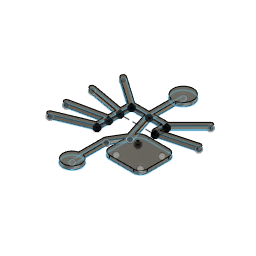
2023_04_27_Conductive Pla v3 (Autodesk Fusion 360 design; units mm, degrees)
Autodesk Fusion 360 part; units mm, degrees
note: some values were not read from the file. Chosen so that the rebuilt part matches the saved one: which bodies a step acts on. Set by a fixed rule: which sketch regions a step uses.
sketch "Sketch1" plane through (0, 0, 0) normal (0, 0, 1) x (1, 0, 0)
  line L0 (0, 0) -> (1.75, 0)
  line L1 (1.75, 0) -> (1.75, 100)
  line L2 (1.75, 100) -> (0, 100)
  line L3 (0, 100) -> (0, 0)
  line L4 (4.7368, 100) -> (4.7368, 0)
  line L5 (4.7368, 0) -> (6.4868, 0)
  line L6 (6.4868, 100) -> (4.7368, 100)
  line L7 (6.4868, 0) -> (6.4868, 100)
  line L8 (9.4737, 100) -> (9.4737, 0)
  line L9 (9.4737, 0) -> (11.2237, 0)
  line L10 (11.2237, 100) -> (9.4737, 100)
  line L11 (11.2237, 0) -> (11.2237, 100)
  line L12 (14.2105, 100) -> (14.2105, 0)
  line L13 (14.2105, 0) -> (15.9605, 0)
  line L14 (15.9605, 100) -> (14.2105, 100)
  line L15 (15.9605, 0) -> (15.9605, 100)
  line L16 (18.9474, 100) -> (18.9474, 0)
  line L17 (18.9474, 0) -> (20.6974, 0)
  line L18 (20.6974, 100) -> (18.9474, 100)
  line L19 (20.6974, 0) -> (20.6974, 100)
  line L20 (23.6842, 100) -> (23.6842, 0)
  line L21 (23.6842, 0) -> (25.4342, 0)
  line L22 (25.4342, 100) -> (23.6842, 100)
  line L23 (25.4342, 0) -> (25.4342, 100)
  line L24 (28.4211, 100) -> (28.4211, 0)
  line L25 (28.4211, 0) -> (30.1711, 0)
  line L26 (30.1711, 100) -> (28.4211, 100)
  line L27 (30.1711, 0) -> (30.1711, 100)
  line L28 (33.1579, 100) -> (33.1579, 0)
  line L29 (33.1579, 0) -> (34.9079, 0)
  line L30 (34.9079, 100) -> (33.1579, 100)
  line L31 (34.9079, 0) -> (34.9079, 100)
  line L32 (37.8947, 100) -> (37.8947, 0)
  line L33 (37.8947, 0) -> (39.6447, 0)
  line L34 (39.6447, 100) -> (37.8947, 100)
  line L35 (39.6447, 0) -> (39.6447, 100)
  line L36 (42.6316, 100) -> (42.6316, 0)
  line L37 (42.6316, 0) -> (44.3816, 0)
  line L38 (44.3816, 100) -> (42.6316, 100)
  line L39 (44.3816, 0) -> (44.3816, 100)
  line L40 (47.3684, 100) -> (47.3684, 0)
  line L41 (47.3684, 0) -> (49.1184, 0)
  line L42 (49.1184, 100) -> (47.3684, 100)
  line L43 (49.1184, 0) -> (49.1184, 100)
  line L44 (52.1053, 100) -> (52.1053, 0)
  line L45 (52.1053, 0) -> (53.8553, 0)
  line L46 (53.8553, 100) -> (52.1053, 100)
  line L47 (53.8553, 0) -> (53.8553, 100)
  line L48 (56.8421, 100) -> (56.8421, 0)
  line L49 (56.8421, 0) -> (58.5921, 0)
  line L50 (58.5921, 100) -> (56.8421, 100)
  line L51 (58.5921, 0) -> (58.5921, 100)
  line L52 (61.5789, 100) -> (61.5789, 0)
  line L53 (61.5789, 0) -> (63.3289, 0)
  line L54 (63.3289, 100) -> (61.5789, 100)
  line L55 (63.3289, 0) -> (63.3289, 100)
  line L56 (66.3158, 100) -> (66.3158, 0)
  line L57 (66.3158, 0) -> (68.0658, 0)
  line L58 (68.0658, 100) -> (66.3158, 100)
  line L59 (68.0658, 0) -> (68.0658, 100)
  line L60 (71.0526, 100) -> (71.0526, 0)
  line L61 (71.0526, 0) -> (72.8026, 0)
  line L62 (72.8026, 100) -> (71.0526, 100)
  line L63 (72.8026, 0) -> (72.8026, 100)
  line L64 (75.7895, 100) -> (75.7895, 0)
  line L65 (75.7895, 0) -> (77.5395, 0)
  line L66 (77.5395, 100) -> (75.7895, 100)
  line L67 (77.5395, 0) -> (77.5395, 100)
  line L68 (80.5263, 100) -> (80.5263, 0)
  line L69 (80.5263, 0) -> (82.2763, 0)
  line L70 (82.2763, 100) -> (80.5263, 100)
  line L71 (82.2763, 0) -> (82.2763, 100)
  line L72 (85.2632, 100) -> (85.2632, 0)
  line L73 (85.2632, 0) -> (87.0132, 0)
  line L74 (87.0132, 100) -> (85.2632, 100)
  line L75 (87.0132, 0) -> (87.0132, 100)
  line L76 (90, 100) -> (90, 0)
  line L77 (90, 0) -> (91.75, 0)
  line L78 (91.75, 100) -> (90, 100)
  line L79 (91.75, 0) -> (91.75, 100)
  line L80 (0, 100) -> (6.4868, 100)
  line L81 (6.4868, 100) -> (6.4868, 97.0952)
  line L82 (6.4868, 97.0952) -> (0, 97.0952)
  line L83 (0, 97.0952) -> (0, 100)
  line L84 (4.7368, 0) -> (11.2237, 0)
  line L85 (11.2237, 0) -> (11.2237, 2.7697)
  line L86 (11.2237, 2.7697) -> (4.7368, 2.7697)
  line L87 (4.7368, 2.7697) -> (4.7368, 0)
  line L88 (9.5, 100) -> (15.9868, 100)
  line L89 (15.9868, 100) -> (15.9868, 97.0952)
  line L90 (9.5, 97.0952) -> (9.5, 100)
  line L91 (15.9868, 97.0952) -> (9.5, 97.0952)
  line L92 (14.2368, 0) -> (20.7237, 0)
  line L93 (20.7237, 0) -> (20.7237, 2.7697)
  line L94 (14.2368, 2.7697) -> (14.2368, 0)
  line L95 (20.7237, 2.7697) -> (14.2368, 2.7697)
  line L96 (19, 100) -> (25.4868, 100)
  line L97 (25.4868, 100) -> (25.4868, 97.0952)
  line L98 (19, 97.0952) -> (19, 100)
  line L99 (25.4868, 97.0952) -> (19, 97.0952)
  line L100 (23.7368, 0) -> (30.2237, 0)
  line L101 (30.2237, 0) -> (30.2237, 2.7697)
  line L102 (23.7368, 2.7697) -> (23.7368, 0)
  line L103 (30.2237, 2.7697) -> (23.7368, 2.7697)
  line L104 (28.5, 100) -> (34.9868, 100)
  line L105 (34.9868, 100) -> (34.9868, 97.0952)
  line L106 (28.5, 97.0952) -> (28.5, 100)
  line L107 (34.9868, 97.0952) -> (28.5, 97.0952)
  line L108 (33.2368, 0) -> (39.7237, 0)
  line L109 (39.7237, 0) -> (39.7237, 2.7697)
  line L110 (33.2368, 2.7697) -> (33.2368, 0)
  line L111 (39.7237, 2.7697) -> (33.2368, 2.7697)
  line L112 (38, 100) -> (44.4868, 100)
  line L113 (44.4868, 100) -> (44.4868, 97.0952)
  line L114 (38, 97.0952) -> (38, 100)
  line L115 (44.4868, 97.0952) -> (38, 97.0952)
  line L116 (42.7368, 0) -> (49.2237, 0)
  line L117 (49.2237, 0) -> (49.2237, 2.7697)
  line L118 (42.7368, 2.7697) -> (42.7368, 0)
  line L119 (49.2237, 2.7697) -> (42.7368, 2.7697)
  line L120 (47.5, 100) -> (53.9868, 100)
  line L121 (53.9868, 100) -> (53.9868, 97.0952)
  line L122 (47.5, 97.0952) -> (47.5, 100)
  line L123 (53.9868, 97.0952) -> (47.5, 97.0952)
  line L124 (52.2368, 0) -> (58.7237, 0)
  line L125 (58.7237, 0) -> (58.7237, 2.7697)
  line L126 (52.2368, 2.7697) -> (52.2368, 0)
  line L127 (58.7237, 2.7697) -> (52.2368, 2.7697)
  line L128 (57, 100) -> (63.4868, 100)
  line L129 (63.4868, 100) -> (63.4868, 97.0952)
  line L130 (57, 97.0952) -> (57, 100)
  line L131 (63.4868, 97.0952) -> (57, 97.0952)
  line L132 (61.7368, 0) -> (68.2237, 0)
  line L133 (68.2237, 0) -> (68.2237, 2.7697)
  line L134 (61.7368, 2.7697) -> (61.7368, 0)
  line L135 (68.2237, 2.7697) -> (61.7368, 2.7697)
  line L136 (66.5, 100) -> (72.9868, 100)
  line L137 (72.9868, 100) -> (72.9868, 97.0952)
  line L138 (66.5, 97.0952) -> (66.5, 100)
  line L139 (72.9868, 97.0952) -> (66.5, 97.0952)
  line L140 (71.2368, 0) -> (77.7237, 0)
  line L141 (77.7237, 0) -> (77.7237, 2.7697)
  line L142 (71.2368, 2.7697) -> (71.2368, 0)
  line L143 (77.7237, 2.7697) -> (71.2368, 2.7697)
  line L144 (76, 100) -> (82.4868, 100)
  line L145 (82.4868, 100) -> (82.4868, 97.0952)
  line L146 (76, 97.0952) -> (76, 100)
  line L147 (82.4868, 97.0952) -> (76, 97.0952)
  line L148 (80.7368, 0) -> (87.2237, 0)
  line L149 (87.2237, 0) -> (87.2237, 2.7697)
  line L150 (80.7368, 2.7697) -> (80.7368, 0)
  line L151 (87.2237, 2.7697) -> (80.7368, 2.7697)
  line L152 (85.5, 100) -> (91.9868, 100)
  line L153 (91.9868, 100) -> (91.9868, 97.0952)
  line L154 (85.5, 97.0952) -> (85.5, 100)
  line L155 (91.9868, 97.0952) -> (85.5, 97.0952)
  line L156 (90.2368, 0) -> (96.7237, 0)
  line L157 (96.7237, 0) -> (96.7237, 2.7697)
  line L158 (90.2368, 2.7697) -> (90.2368, 0)
  line L159 (96.7237, 2.7697) -> (90.2368, 2.7697)
  line L160 (109.2368, 2.7697) -> (109.2368, 0)
  line L161 (182.0132, 0) -> (182.0132, 100)
  line L162 (170.7895, 100) -> (170.7895, 0)
  line L163 (147.2368, 2.7697) -> (147.2368, 0)
  line L164 (134.6447, 100) -> (132.8947, 100)
  line L165 (153.5921, 0) -> (153.5921, 100)
  line L166 (125.2237, 0) -> (125.2237, 2.7697)
  line L167 (147.2368, 0) -> (153.7237, 0)
  line L168 (166.0526, 100) -> (166.0526, 0)
  line L169 (180.2632, 100) -> (180.2632, 0)
  line L170 (115.6974, 0) -> (115.6974, 100)
  line L171 (185, 0) -> (186.75, 0)
  line L172 (118.7368, 0) -> (125.2237, 0)
  line L173 (96.75, 0) -> (96.75, 100)
  line L174 (120.4342, 0) -> (120.4342, 100)
  line L175 (115.6974, 100) -> (113.9474, 100)
  line L176 (128.2368, 2.7697) -> (128.2368, 0)
  line L177 (139.4868, 97.0952) -> (133, 97.0952)
  line L178 (109.2368, 0) -> (115.7237, 0)
  line L179 (128.1579, 100) -> (128.1579, 0)
  line L180 (161.3158, 100) -> (161.3158, 0)
  line L181 (144.1184, 0) -> (144.1184, 100)
  line L182 (166.2368, 0) -> (172.7237, 0)
  line L183 (170.7895, 0) -> (172.5395, 0)
  line L184 (113.9474, 0) -> (115.6974, 0)
  line L185 (134.7237, 2.7697) -> (128.2368, 2.7697)
  line L186 (163.0658, 0) -> (163.0658, 100)
  line L187 (148.8553, 0) -> (148.8553, 100)
  line L188 (172.7237, 0) -> (172.7237, 2.7697)
  line L189 (99.7368, 0) -> (101.4868, 0)
  line L190 (144.2237, 0) -> (144.2237, 2.7697)
  line L191 (137.6316, 0) -> (139.3816, 0)
  line L192 (137.7368, 2.7697) -> (137.7368, 0)
  line L193 (153.7237, 0) -> (153.7237, 2.7697)
  line L194 (175.5263, 0) -> (177.2763, 0)
  line L195 (120.4868, 100) -> (120.4868, 97.0952)
  line L196 (139.3816, 0) -> (139.3816, 100)
  line L197 (186.75, 0) -> (186.75, 100)
  line L198 (177.2763, 0) -> (177.2763, 100)
  line L199 (156.5789, 100) -> (156.5789, 0)
  line L200 (125.1711, 0) -> (125.1711, 100)
  line L201 (95, 97.0952) -> (95, 100)
  line L202 (123.4211, 100) -> (123.4211, 0)
  line L203 (158.3289, 0) -> (158.3289, 100)
  line L204 (104.4737, 0) -> (106.2237, 0)
  line L205 (156.5789, 0) -> (158.3289, 0)
  line L206 (147.1053, 100) -> (147.1053, 0)
  line L207 (123.4211, 0) -> (125.1711, 0)
  line L208 (175.7368, 2.7697) -> (175.7368, 0)
  line L209 (175.7368, 0) -> (182.2237, 0)
  line L210 (175.5263, 100) -> (175.5263, 0)
  line L211 (182.2237, 0) -> (182.2237, 2.7697)
  line L212 (104.5, 100) -> (110.9868, 100)
  line L213 (180.2632, 0) -> (182.0132, 0)
  line L214 (128.1579, 0) -> (129.9079, 0)
  line L215 (137.6316, 100) -> (137.6316, 0)
  line L216 (177.4868, 97.0952) -> (171, 97.0952)
  line L217 (110.9868, 97.0952) -> (104.5, 97.0952)
  line L218 (95, 0) -> (96.75, 0)
  line L219 (99.7368, 0) -> (106.2237, 0)
  line L220 (161.5, 100) -> (167.9868, 100)
  line L221 (110.9868, 100) -> (110.9868, 97.0952)
  line L222 (156.7368, 2.7697) -> (156.7368, 0)
  line L223 (163.2237, 2.7697) -> (156.7368, 2.7697)
  line L224 (153.7237, 2.7697) -> (147.2368, 2.7697)
  line L225 (142.3684, 0) -> (144.1184, 0)
  line L226 (185, 100) -> (185, 0)
  line L227 (104.4737, 100) -> (104.4737, 0)
  line L228 (99.7368, 100) -> (99.7368, 0)
  line L229 (166.0526, 0) -> (167.8026, 0)
  line L230 (180.5, 97.0952) -> (180.5, 100)
  line L231 (156.7368, 0) -> (163.2237, 0)
  line L232 (172.5395, 0) -> (172.5395, 100)
  line L233 (134.7237, 0) -> (134.7237, 2.7697)
  line L234 (185.2368, 0) -> (191.7237, 0)
  line L235 (120.4868, 97.0952) -> (114, 97.0952)
  line L236 (185.2368, 2.7697) -> (185.2368, 0)
  line L237 (172.7237, 2.7697) -> (166.2368, 2.7697)
  line L238 (167.9868, 100) -> (167.9868, 97.0952)
  line L239 (142.3684, 100) -> (142.3684, 0)
  line L240 (101.4868, 100) -> (99.7368, 100)
  line L241 (151.8421, 100) -> (151.8421, 0)
  line L242 (147.1053, 0) -> (148.8553, 0)
  line L243 (133, 100) -> (139.4868, 100)
  line L244 (167.9868, 97.0952) -> (161.5, 97.0952)
  line L245 (163.2237, 0) -> (163.2237, 2.7697)
  line L246 (132.8947, 0) -> (134.6447, 0)
  line L247 (129.9868, 100) -> (129.9868, 97.0952)
  line L248 (118.7368, 2.7697) -> (118.7368, 0)
  line L249 (151.8421, 0) -> (153.5921, 0)
  line L250 (109.2105, 100) -> (109.2105, 0)
  line L251 (158.3289, 100) -> (156.5789, 100)
  line L252 (132.8947, 100) -> (132.8947, 0)
  line L253 (118.6842, 0) -> (120.4342, 0)
  line L254 (95, 100) -> (95, 0)
  line L255 (115.7237, 0) -> (115.7237, 2.7697)
  line L256 (118.6842, 100) -> (118.6842, 0)
  line L257 (106.2237, 0) -> (106.2237, 2.7697)
  line L258 (125.1711, 100) -> (123.4211, 100)
  line L259 (113.9474, 100) -> (113.9474, 0)
  line L260 (101.4868, 0) -> (101.4868, 100)
  line L261 (128.2368, 0) -> (134.7237, 0)
  line L262 (106.2237, 0) -> (106.2237, 100)
  line L263 (134.6447, 0) -> (134.6447, 100)
  line L264 (110.9605, 0) -> (110.9605, 100)
  line L265 (96.75, 100) -> (95, 100)
  line L266 (106.2237, 100) -> (104.4737, 100)
  line L267 (99.7368, 2.7697) -> (99.7368, 0)
  line L268 (110.9605, 100) -> (109.2105, 100)
  line L269 (129.9079, 100) -> (128.1579, 100)
  line L270 (158.4868, 97.0952) -> (152, 97.0952)
  line L271 (142.5, 100) -> (148.9868, 100)
  line L272 (180.5, 100) -> (186.9868, 100)
  line L273 (182.0132, 100) -> (180.2632, 100)
  line L274 (166.2368, 2.7697) -> (166.2368, 0)
  line L275 (144.1184, 100) -> (142.3684, 100)
  line L276 (139.4868, 100) -> (139.4868, 97.0952)
  line L277 (106.2237, 2.7697) -> (99.7368, 2.7697)
  line L278 (104.5, 97.0952) -> (104.5, 100)
  line L279 (167.8026, 100) -> (166.0526, 100)
  line L280 (191.7237, 2.7697) -> (185.2368, 2.7697)
  line L281 (182.2237, 2.7697) -> (175.7368, 2.7697)
  line L282 (161.5, 97.0952) -> (161.5, 100)
  line L283 (144.2237, 2.7697) -> (137.7368, 2.7697)
  line L284 (137.7368, 0) -> (144.2237, 0)
  line L285 (142.5, 97.0952) -> (142.5, 100)
  line L286 (133, 97.0952) -> (133, 100)
  line L287 (186.9868, 97.0952) -> (180.5, 97.0952)
  line L288 (177.4868, 100) -> (177.4868, 97.0952)
  line L289 (171, 100) -> (177.4868, 100)
  line L290 (123.5, 100) -> (129.9868, 100)
  line L291 (114, 100) -> (120.4868, 100)
  line L292 (158.4868, 100) -> (158.4868, 97.0952)
  line L293 (148.9868, 97.0952) -> (142.5, 97.0952)
  line L294 (120.4342, 100) -> (118.6842, 100)
  line L295 (129.9868, 97.0952) -> (123.5, 97.0952)
  line L296 (101.4868, 100) -> (101.4868, 97.0952)
  line L297 (114, 97.0952) -> (114, 100)
  line L298 (167.8026, 0) -> (167.8026, 100)
  line L299 (161.3158, 0) -> (163.0658, 0)
  line L300 (186.75, 100) -> (185, 100)
  line L301 (95, 100) -> (101.4868, 100)
  line L302 (101.4868, 97.0952) -> (95, 97.0952)
  line L303 (148.8553, 100) -> (147.1053, 100)
  line L304 (153.5921, 100) -> (151.8421, 100)
  line L305 (172.5395, 100) -> (170.7895, 100)
  line L306 (123.5, 97.0952) -> (123.5, 100)
  line L307 (115.7237, 2.7697) -> (109.2368, 2.7697)
  line L308 (191.7237, 0) -> (191.7237, 2.7697)
  line L309 (177.2763, 100) -> (175.5263, 100)
  line L310 (148.9868, 100) -> (148.9868, 97.0952)
  line L311 (125.2237, 2.7697) -> (118.7368, 2.7697)
  line L312 (139.3816, 100) -> (137.6316, 100)
  line L313 (152, 100) -> (158.4868, 100)
  line L314 (109.2105, 0) -> (110.9605, 0)
  line L315 (129.9079, 0) -> (129.9079, 100)
  line L316 (186.9868, 100) -> (186.9868, 97.0952)
  line L317 (152, 97.0952) -> (152, 100)
  line L318 (171, 97.0952) -> (171, 100)
  line L319 (163.0658, 100) -> (161.3158, 100)
  point P0 (95, 0)
  dimension "d1" = 1.75
  dimension "d2" = 100
  dimension "d5" = 90
  dimension "d6" = 0
  dimension "d9" = 9.5
  dimension "d10" = 0
  dimension "d13" = 90
  dimension "d14" = 0
  dimension "d17" = 9.5
  dimension "d18" = 0
  dimension "d19" = 1.75
  dimension "d20" = 100
  constraint horizontal L0
  constraint vertical L1
  constraint horizontal L2
  constraint vertical L3
  constraint coincident L0.start L3.end
  constraint horizontal L80
  constraint vertical L81
  constraint horizontal L82
  constraint vertical L83
  constraint coincident L7 L81.end
  constraint horizontal L84
  constraint vertical L85
  constraint horizontal L86
  constraint vertical L87
  constraint coincident L11 L85.end
  constraint horizontal L218
  constraint vertical L173
  constraint horizontal L265
  constraint vertical L254
  constraint coincident P0 L218.start
  constraint horizontal L301
  constraint vertical L296
  constraint horizontal L302
  constraint vertical L201
  constraint coincident L296.end L260
  constraint horizontal L219
  constraint vertical L257
  constraint horizontal L277
  constraint vertical L267
  constraint coincident L257.end L262
  measures "d1" distance of L0.start L0.end
  measures "d2" distance of L0.start L2.end
  measures "d19" distance of P0 L173.start
  measures "d20" distance of L201.end P0
sketch "Sketch2" plane through (0, 0, 0) normal (0, 0, 1) x (1, 0, 0)
  circle A0 centre (20, 130) radius 20
  line L0 (50, 150) -> (100, 150)
  line L1 (100, 150) -> (100, 120)
  line L2 (100, 120) -> (50, 120)
  line L3 (50, 120) -> (50, 150)
  constraint horizontal L0
  constraint vertical L1
  constraint horizontal L2
  constraint vertical L3
extrude "Extrude1" add sketch "Sketch1" sketch "Sketch2" along normal blind 2 of sketch 2 makes body 1 at (66.6667, 140, 0) makes body 2 at (89.0833, 99.0317, 0) makes body 3 at (18.0183, 116.8525, 0)
sketch "Sketch3" plane through (0, 0, 0) normal (0, 0, 1) x (1, 0, 0)
  line L0 (0, 0) -> (0, 5.08) construction
  line L1 (0, 5.08) -> (0, 10.16) construction
  line L2 (0, 10.16) -> (0, 15.24) construction
  line L3 (0, 15.24) -> (15.5, 15.24) construction
  line L4 (0, 10.16) -> (15.5, 10.16) construction
  circle A0 centre (0, 0) radius 0.3
  circle A1 centre (0, 5.08) radius 0.3
  circle A2 centre (0, 10.16) radius 0.3
  circle A3 centre (0, 15.24) radius 0.3
  circle A4 centre (15.5, 15.24) radius 0.3
  circle A5 centre (15.5, 10.16) radius 0.3
  line L5 (1, 0) -> (1, 15.24)
  arc A6 (1, 15.24) -> (-1, 15.24) centre (0, 15.24) ccw
  line L6 (-1, 15.24) -> (-1, 0)
  arc A7 (-1, 0) -> (1, 0) centre (0, 0) ccw
  line L7 (0, 0) -> (0, 15.24) construction
  line L8 (14.5, 15.24) -> (14.5, 10.16)
  arc A8 (14.5, 10.16) -> (16.5, 10.16) centre (15.5, 10.16) ccw
  line L9 (16.5, 10.16) -> (16.5, 15.24)
  arc A9 (16.5, 15.24) -> (14.5, 15.24) centre (15.5, 15.24) ccw
  line L10 (15.5, 15.24) -> (15.5, 10.16) construction
  line L11 (0, 14.24) -> (15.5, 14.24)
  arc A10 (15.5, 14.24) -> (15.5, 16.24) centre (15.5, 15.24) ccw
  line L12 (15.5, 16.24) -> (0, 16.24)
  arc A11 (0, 16.24) -> (0, 14.24) centre (0, 15.24) ccw
  line L13 (0, 15.24) -> (15.5, 15.24) construction
  line L14 (16.2071, 14.5329) -> (25.838, 24.1638)
  arc A12 (25.838, 24.1638) -> (24.4238, 25.578) centre (25.1309, 24.8709) ccw
  line L15 (24.4238, 25.578) -> (14.7929, 15.9471)
  arc A13 (14.7929, 15.9471) -> (16.2071, 14.5329) centre (15.5, 15.24) ccw
  line L16 (15.5, 15.24) -> (25.1309, 24.8709) construction
  line L17 (15.5, 10.16) -> (15.5, 2.54) construction
  circle A14 centre (15.5, 2.54) radius 0.3
  line L18 (15.5, 6.35) -> (25.3285, 6.35)
  line L19 (28.3285, 3.35) -> (28.3285, -6.1848)
  line L20 (25.3285, -9.1848) -> (14.7009, -9.1848)
  line L21 (11.7009, -6.1848) -> (11.7009, 2.8277)
  line L22 (15.7604, 9.1945) -> (30.8902, 13.2745)
  arc A15 (30.8902, 13.2745) -> (30.3695, 15.2055) centre (30.6299, 14.24) ccw
  line L23 (30.3695, 15.2055) -> (15.2396, 11.1255)
  arc A16 (15.2396, 11.1255) -> (15.7604, 9.1945) centre (15.5, 10.16) ccw
  line L24 (15.5, 10.16) -> (30.6299, 14.24) construction
  line L25 (0.5736, 16.0592) -> (-11.7137, 24.6628)
  arc A17 (-11.7137, 24.6628) -> (-12.8609, 23.0245) centre (-12.2873, 23.8436) ccw
  line L26 (-12.8609, 23.0245) -> (-0.5736, 14.4208)
  arc A18 (-0.5736, 14.4208) -> (0.5736, 16.0592) centre (0, 15.24) ccw
  line L27 (0, 15.24) -> (-12.2873, 23.8436) construction
  line L28 (0.1792, 11.1438) -> (-14.8753, 13.8861)
  arc A19 (-14.8753, 13.8861) -> (-15.2337, 11.9184) centre (-15.0545, 12.9023) ccw
  line L29 (-15.2337, 11.9184) -> (-0.1792, 9.1762)
  arc A20 (-0.1792, 9.1762) -> (0.1792, 11.1438) centre (0, 10.16) ccw
  line L30 (0, 10.16) -> (-15.0545, 12.9023) construction
  line L31 (-0.2065, 6.0584) -> (-15.4865, 2.8334)
  arc A21 (-15.4865, 2.8334) -> (-15.0734, 0.8765) centre (-15.2799, 1.855) ccw
  line L32 (-15.0734, 0.8765) -> (0.2065, 4.1016)
  arc A22 (0.2065, 4.1016) -> (-0.2065, 6.0584) centre (0, 5.08) ccw
  line L33 (0, 5.08) -> (-15.2799, 1.855) construction
  line L34 (-0.3859, 0.9226) -> (-15.0145, -5.1958)
  arc A23 (-15.0145, -5.1958) -> (-14.2428, -7.041) centre (-14.6286, -6.1184) ccw
  line L35 (-14.2428, -7.041) -> (0.3859, -0.9226)
  arc A24 (0.3859, -0.9226) -> (-0.3859, 0.9226) centre (0, 0) ccw
  line L36 (0, 0) -> (-14.6286, -6.1184) construction
  arc A25 (15.5, 6.35) -> (11.7009, 2.2523) centre (15.5, 2.54) ccw
  arc A26 (28.3285, 3.35) -> (25.3285, 6.35) centre (25.3285, 3.35) ccw
  arc A27 (25.3285, -9.1848) -> (28.3285, -6.1848) centre (25.3285, -6.1848) ccw
  arc A28 (11.7009, -6.1848) -> (14.7009, -9.1848) centre (14.7009, -6.1848) ccw
  line L37 (12.6538, 3.131) -> (8.7029, 15.5433)
  arc A29 (8.7029, 15.5433) -> (6.7971, 14.9367) centre (7.75, 15.24) ccw
  line L38 (6.7971, 14.9367) -> (10.748, 2.5244)
  arc A30 (10.748, 2.5244) -> (12.6538, 3.131) centre (11.7009, 2.8277) ccw
  line L39 (11.7009, 2.8277) -> (7.75, 15.24) construction
  line L40 (8.75, 15.24) -> (8.75, 30.24)
  arc A31 (8.75, 30.24) -> (6.75, 30.24) centre (7.75, 30.24) ccw
  line L41 (6.75, 30.24) -> (6.75, 15.24)
  arc A32 (6.75, 15.24) -> (8.75, 15.24) centre (7.75, 15.24) ccw
  line L42 (7.75, 15.24) -> (7.75, 30.24) construction
  line L43 (10.8466, 3.3474) -> (6.8957, -3.1467)
  arc A33 (6.8957, -3.1467) -> (8.6043, -4.1862) centre (7.75, -3.6665) ccw
  line L44 (8.6043, -4.1862) -> (12.5552, 2.308)
  arc A34 (12.5552, 2.308) -> (10.8466, 3.3474) centre (11.7009, 2.8277) ccw
  line L45 (11.7009, 2.8277) -> (7.75, -3.6665) construction
  line L46 (6.75, -3.6665) -> (6.75, -18.6665)
  arc A35 (6.75, -18.6665) -> (8.75, -18.6665) centre (7.75, -18.6665) ccw
  line L47 (8.75, -18.6665) -> (8.75, -3.6665)
  arc A36 (8.75, -3.6665) -> (6.75, -3.6665) centre (7.75, -3.6665) ccw
  line L48 (7.75, -3.6665) -> (7.75, -18.6665) construction
  circle A37 centre (7.75, 30.24) radius 4.4272
  circle A38 centre (7.75, -18.6665) radius 4
  dimension "d23" = 5.08
  dimension "d24" = 5.08
  dimension "d25" = 5.08
  dimension "d26" = 15.5
  dimension "d27" = 15.5
  dimension "d28" = 0.6
  dimension "d29" = 2
  dimension "d30" = 2
  dimension "d31" = 7.62
  dimension "d32" = 0.6
  dimension "d33" = 2
  dimension "d34" = 2
  dimension "d35" = 2
  dimension "d36" = 2
  dimension "d37" = 2
  dimension "d38" = 3
  dimension "d39" = 2
  dimension "d40" = 2
  dimension "d41" = 2
  dimension "d42" = 2
  dimension "d43" = 8
  constraint coincident L0.start A0.centre
  constraint vertical L0
  constraint vertical L1
  constraint parallel L1 L2
  constraint perpendicular L2 L3
  constraint perpendicular L2 L4
  constraint coincident L0.end L1.start
  constraint coincident L1.end L2.start
  constraint coincident L2.end L3.start
  constraint coincident L3.end A4.centre
  constraint coincident L4.end A5.centre
  constraint equal A0 A1
  constraint equal A0 A2
  constraint equal A0 A5
  constraint equal A0 A3
  constraint equal A0 A4
  constraint tangent L5 A6
  constraint tangent A6 L6
  constraint parallel L5 L6
  constraint tangent L6 A7
  constraint tangent L5 A7
  constraint perpendicular L3 L7
  constraint tangent L8 A8
  constraint tangent A8 L9
  constraint parallel L8 L9
  constraint tangent L9 A9
  constraint tangent L8 A9
  constraint perpendicular L3 L10
  constraint tangent L11 A10
  constraint tangent A10 L12
  constraint parallel L11 L12
  constraint tangent L12 A11
  constraint tangent L11 A11
  constraint perpendicular L10 L13
  constraint tangent L14 A12
  constraint tangent A12 L15
  constraint parallel L14 L15
  constraint tangent L15 A13
  constraint tangent L14 A13
  constraint parallel L10 L17
  constraint coincident L17.end A14.centre
  constraint concentric A14 A25
  constraint horizontal L18
  constraint vertical L19
  constraint horizontal L20
  constraint vertical L21
  constraint tangent L22 A15
  constraint tangent A15 L23
  constraint parallel L22 L23
  constraint tangent L23 A16
  constraint tangent L22 A16
  constraint tangent L25 A17
  constraint tangent A17 L26
  constraint parallel L25 L26
  constraint tangent L26 A18
  constraint tangent L25 A18
  constraint tangent L28 A19
  constraint tangent A19 L29
  constraint parallel L28 L29
  constraint tangent L29 A20
  constraint tangent L28 A20
  constraint tangent L31 A21
  constraint tangent A21 L32
  constraint parallel L31 L32
  constraint tangent L32 A22
  constraint tangent L31 A22
  constraint tangent L34 A23
  constraint tangent A23 L35
  constraint parallel L34 L35
  constraint tangent L35 A24
  constraint tangent L34 A24
  constraint coincident L21.end A25
  constraint coincident L17 L18.start
  constraint coincident L21 A25.end
  constraint tangent L18 A26
  constraint tangent L19 A26
  constraint tangent L20 A27
  constraint tangent L19 A27
  constraint equal A26 A27
  constraint tangent L20 A28
  constraint tangent L21 A28
  constraint equal A26 A28
  constraint tangent L37 A29
  constraint tangent A29 L38
  constraint parallel L37 L38
  constraint tangent L38 A30
  constraint tangent L37 A30
  constraint midpoint L3 A29.centre
  constraint coincident L21.end A30.centre
  constraint tangent L40 A31
  constraint tangent A31 L41
  constraint parallel L40 L41
  constraint tangent L41 A32
  constraint tangent L40 A32
  constraint perpendicular L12 L42
  constraint coincident A29.centre L39.end
  constraint tangent L43 A33
  constraint tangent A33 L44
  constraint parallel L43 L44
  constraint tangent L44 A34
  constraint tangent L43 A34
  constraint tangent L46 A35
  constraint tangent A35 L47
  constraint parallel L46 L47
  constraint tangent L47 A36
  constraint tangent L46 A36
  constraint vertical L48
  constraint coincident A33.centre L45.end
  constraint concentric A31 A37
  constraint concentric A35 A38
  measures "d23" distance of L0.start L0.end
  measures "d24" distance of L0.end L1.end
  measures "d25" distance of L1.end L2.end
  measures "d26" distance of L2.end L3.end
  measures "d27" distance of L1.end L4.end
  measures "d28" diameter of A0
  measures "d29" diameter of A8
  measures "d30" diameter of A12
  measures "d31" distance of L4.end L17.end
  measures "d32" diameter of A14
  measures "d33" diameter of A15
  measures "d34" diameter of A17
  measures "d35" diameter of A19
  measures "d36" diameter of A21
  measures "d37" diameter of A23
  measures "d38" radius of A26
  measures "d39" diameter of A29
  measures "d40" diameter of A31
  measures "d41" diameter of A33
  measures "d42" diameter of A35
  measures "d43" diameter of A38
sketch "Sketch4" plane through (0, 0, 0) normal (1, 0, 0) x (0, 1, 0)
extrude "Extrude2" add sketch "Sketch3" along normal blind 1.5 separate body contours A0 | A1 | A2 | A3 | A4 | A5 | L5 L6 L32 A22 L34 A24 | L6 A7 L34 A24 | L5 L6 L29 A20 L31 A22 | L6 L31 L32 A22 | L6 A7 L34 A23 L35 | L5 L6 L11 A11 L26 A18 L28 A20 | L6 L28 L29 A20 | L5 L11 A18 | L5 A6 L11 L12 L25 A18 A29 L38 L41 A32 | L6 L31 A21 L32 | A6 A11 A18 | L11 L38 A32 | L11 A25 L37 L38 L43 A34 | L6 L28 A19 L29 | A6 L12 L25 | L6 A11 L26 | L11 L37 L40 A32 | L37 A29 L40 A32 | L21 A25 L38 A30 L43 A34 | L21 L38 A30 L43 L44 L47 A36 | A6 L6 L12 A11 L25 A17 L26 | L8 A9 L11 L12 L15 A13 L37 L40 | L12 A29 L41 | A33 L44 L47 A36 | L12 L40 L41 A37 | L8 L9 L11 A10 L14 A13 L23 A16 | L8 L11 A13 | A25 L37 A34 | L18 L19 L20 L21 A25 A26 A27 A28 L37 A30 L44 A34 | L12 L37 A29 L40 | L21 A30 L44 | L21 A25 A30 A34 | A33 L44 L46 L47 A38 | L40 A31 L41 A37 | L40 A31 L41 A37 | A9 A10 A13 | A8 L9 L23 A16 | L21 A25 | L46 A35 L47 A38 | L46 A35 L47 A38 | A9 L12 L15 | A8 L9 L22 A15 L23 | L9 A10 L14 | L9 A9 A10 L12 L14 A12 L15 | A14 makes body 4
extrude "Extrude3" cut sketch "Sketch3" along normal blind 10 contours A0 | A1 | A2 | A3 | A4 | A5 | A14 bodies 4
hidden bodies 1 2 3
equation "d23 = ( 2.54 * 2 ) * 1 mm"
equation "d24 = ( 2.54 * 2 ) * 1 mm"
equation "d25 = ( 2.54 * 2 ) * 1 mm"
equation "d31 = ( 2.54 * 3 ) * 1 mm"
named bodies: "Square", "Long Line", "Circlee"
